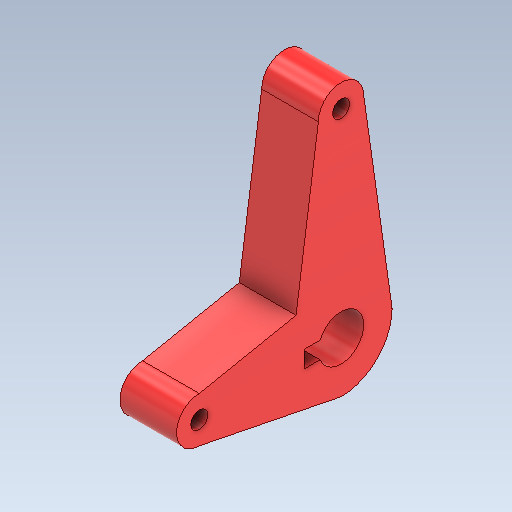
# Autodesk Inventor part: hw3
Saved by Autodesk Inventor 2021 (Build 250183000, 183)
## iProperties
Created: 2022-04-30
Part Number: hw3
Material: Generic
Document SubType Name: Modeling
Designer: authe
Density: 1 g/cm^3
Appearance: Light Red
Author: authe
Autodesk Inventor part; units mm, degrees
ref_plane "YZ Plane" through (0, 0, 0) normal (1, 0, 0) x (0, 1, 0)
ref_plane "XZ Plane" through (0, 0, 0) normal (0, 1, 0) x (-1, 0, 0)
ref_plane "XY Plane" through (0, 0, 0) normal (0, 0, 1) x (1, 0, 0)
sketch "Sketch2" plane through (0, 0, 0) normal (1, 0, 0) x (0, 1, 0)
  circle A0 centre (0, 0) radius 18
  circle A1 centre (0, 0) radius 8
  line L0 (0, 0) -> (70, 0)
  circle A2 centre (70, 0) radius 3
  circle A3 centre (70, 0) radius 8
  line L1 (0, 0) -> (0, 50)
  circle A4 centre (0, 50) radius 3
  circle A5 centre (0, 50) radius 8
  line L2 (70, -8) -> (0, -18)
  line L3 (-8, 50) -> (-18, 0)
  line L4 (70, 8) -> (14.8235, 15.8824)
  line L5 (8, 50) -> (14.8235, 15.8824)
  line L6 (0, 8) -> (0, 13)
  line L7 (0, 13) -> (3, 13)
  line L8 (3, 13) -> (3, 7.4162)
  line L9 (0, 13) -> (-3, 13)
  line L10 (-3, 13) -> (-3, 7.4162)
  dimension "d0" = 36
  dimension "d1" = 16
  dimension "d2" = 70
  dimension "d3" = 6
  dimension "d4" = 16
  dimension "d5" = 50
  dimension "d6" = 6
  dimension "d7" = 16
  dimension "d14" = 5
  dimension "d15" = 3
  dimension "d16" = 3
  constraints: 22 end point, 9 point on circle, 6 centre point, 6 coincident, 3 point on line, 2 perpendicular, 1 horizontal, 1 vertical
  measures "d0" diameter of A0
  measures "d1" diameter of A1
  measures "d2" distance of L0.start L0.end
  measures "d3" diameter of A2
  measures "d4" diameter of A3
  measures "d5" distance of L0.start L1.end
  measures "d6" diameter of A4
  measures "d7" diameter of A5
  measures "d14" distance of L6.start L6.end
  measures "d15" distance of L6.end L7.end
  measures "d16" distance of L6.end L9.end
sketch "Sketch3" plane through (0, 0, 0) normal (1, 0, 0) x (0, 1, 0)
  line L0 (-3, 17.6288) -> (-3, 22.6288)
  line L1 (-3, 22.6288) -> (3, 22.6288)
  point P0 (0, 0)
  constraints: 4 end point, 1 perpendicular
sketch "Sketch4" plane through (0, 0, 0) normal (1, 0, 0) x (0, 1, 0)
  point P0 (0, 0)
extrude "Extrusion1" add sketch "Sketch2" along normal blind 10 and the other way blind 10 contours L3 A0 L1 L9 L10 A1 L0 L2 | L3 A5 L1 A0 | A0 L0 A3 L2 | L1 A5 L5 L4 A3 L0 A0 | A0 L0 A1 L8 L7 L1 | A5 | A3
body "Solid1"
